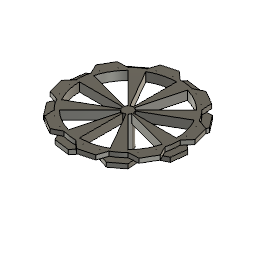
Wheel (Autodesk Fusion 360 design; units mm, degrees)
Autodesk Fusion 360 part; units mm, degrees
sketch "Sketch1" plane through (0, 0, 0) normal (0, 0, 1) x (1, 0, 0)
  circle A0 centre (0, 0) radius 35
  circle A1 centre (0, 0) radius 3.5
  line L0 (0, 0) -> (0, 35)
  line L1 (0, 0) -> (9.0587, 33.8074)
  line L2 (0, 0) -> (35, 0) construction
  line L3 (0, 35) -> (0, 40)
  line L4 (9.0587, 33.8074) -> (10.3528, 38.637)
  line L5 (10.3528, 38.637) -> (0, 40)
  line L6 (-20, 34.641) -> (-28.2843, 28.2843)
  line L7 (-24.7487, 24.7487) -> (-28.2843, 28.2843)
  line L8 (-17.5, 30.3109) -> (-20, 34.641)
  line L9 (0, 0) -> (-24.7487, 24.7487)
  line L10 (0, 0) -> (-17.5, 30.3109)
  line L11 (-38.637, 10.3528) -> (-40, 0)
  line L12 (-35, 0) -> (-40, 0)
  line L13 (-33.8074, 9.0587) -> (-38.637, 10.3528)
  line L14 (0, 0) -> (-35, 0)
  line L15 (0, 0) -> (-33.8074, 9.0587)
  line L16 (-34.641, -20) -> (-28.2843, -28.2843)
  line L17 (-24.7487, -24.7487) -> (-28.2843, -28.2843)
  line L18 (-30.3109, -17.5) -> (-34.641, -20)
  line L19 (0, 0) -> (-24.7487, -24.7487)
  line L20 (0, 0) -> (-30.3109, -17.5)
  line L21 (-10.3528, -38.637) -> (0, -40)
  line L22 (0, -35) -> (0, -40)
  line L23 (-9.0587, -33.8074) -> (-10.3528, -38.637)
  line L24 (0, 0) -> (0, -35)
  line L25 (0, 0) -> (-9.0587, -33.8074)
  line L26 (20, -34.641) -> (28.2843, -28.2843)
  line L27 (24.7487, -24.7487) -> (28.2843, -28.2843)
  line L28 (17.5, -30.3109) -> (20, -34.641)
  line L29 (0, 0) -> (24.7487, -24.7487)
  line L30 (0, 0) -> (17.5, -30.3109)
  line L31 (38.637, -10.3528) -> (40, 0)
  line L32 (35, 0) -> (40, 0)
  line L33 (33.8074, -9.0587) -> (38.637, -10.3528)
  line L34 (0, 0) -> (35, 0)
  line L35 (0, 0) -> (33.8074, -9.0587)
  line L36 (34.641, 20) -> (28.2843, 28.2843)
  line L37 (24.7487, 24.7487) -> (28.2843, 28.2843)
  line L38 (30.3109, 17.5) -> (34.641, 20)
  line L39 (0, 0) -> (24.7487, 24.7487)
  line L40 (0, 0) -> (30.3109, 17.5)
  circle A2 centre (0, 0) radius 32.5
  line L41 (38.637, -10.3528) -> (32.3341, -13.398)
  line L42 (40, 0) -> (34.7, 4.5727)
  line L43 (34.641, 20) -> (32.3375, 13.3899)
  line L44 (28.2843, 28.2843) -> (21.3032, 27.77)
  line L45 (10.3528, 38.637) -> (13.398, 32.3341)
  line L46 (0, 40) -> (-4.5727, 34.7)
  line L47 (-20, 34.641) -> (-13.3899, 32.3375)
  line L48 (-28.2843, 28.2843) -> (-27.77, 21.3032)
  line L49 (-38.637, 10.3528) -> (-32.3341, 13.398)
  line L50 (-40, 0) -> (-34.7, -4.5727)
  line L51 (-34.641, -20) -> (-32.3375, -13.3899)
  line L52 (-28.2843, -28.2843) -> (-21.3032, -27.77)
  line L53 (-10.3528, -38.637) -> (-13.398, -32.3341)
  line L54 (0, -40) -> (4.5727, -34.7)
  line L55 (20, -34.641) -> (13.3899, -32.3375)
  line L56 (28.2843, -28.2843) -> (27.77, -21.3032)
  line L57 (0, 0) -> (13.3939, -32.3358)
  line L58 (0, 0) -> (4.5684, -34.7006)
  line L59 (5.221, -39.6578) -> (15.3073, -36.9552)
  line L60 (15.3073, -36.9552) -> (17.5038, -30.3087)
  line L61 (5.221, -39.6578) -> (-0.0044, -35)
  line L62 (4.5684, -34.7006) -> (5.221, -39.6578)
  line L63 (13.3939, -32.3358) -> (15.3073, -36.9552)
  line L64 (0, 0) -> (24.7487, -24.7487)
  line L65 (0, 0) -> (17.5, -30.3109)
  line L66 (20, -34.641) -> (28.2843, -28.2843)
  line L67 (28.2843, -28.2843) -> (27.77, -21.3032)
  line L68 (20, -34.641) -> (13.3899, -32.3375)
  line L69 (17.5, -30.3109) -> (20, -34.641)
  line L70 (24.7487, -24.7487) -> (28.2843, -28.2843)
  line L71 (0, 0) -> (32.3358, -13.3939)
  line L72 (0, 0) -> (27.7674, -21.3067)
  line L73 (31.7341, -24.3505) -> (36.9552, -15.3073)
  line L74 (36.9552, -15.3073) -> (33.8085, -9.0544)
  line L75 (31.7341, -24.3505) -> (24.7456, -24.7518)
  line L76 (27.7674, -21.3067) -> (31.7341, -24.3505)
  line L77 (32.3358, -13.3939) -> (36.9552, -15.3073)
  line L78 (0, 0) -> (35, 0)
  line L79 (0, 0) -> (33.8074, -9.0587)
  line L80 (38.637, -10.3528) -> (40, 0)
  line L81 (40, 0) -> (34.7, 4.5727)
  line L82 (38.637, -10.3528) -> (32.3341, -13.398)
  line L83 (33.8074, -9.0587) -> (38.637, -10.3528)
  line L84 (35, 0) -> (40, 0)
  line L85 (0, 0) -> (32.3358, 13.3939)
  line L86 (0, 0) -> (34.7006, 4.5684)
  line L87 (39.6578, 5.221) -> (36.9552, 15.3073)
  line L88 (36.9552, 15.3073) -> (30.3087, 17.5038)
  line L89 (39.6578, 5.221) -> (35, -0.0044)
  line L90 (34.7006, 4.5684) -> (39.6578, 5.221)
  line L91 (32.3358, 13.3939) -> (36.9552, 15.3073)
  line L92 (0, 0) -> (24.7487, 24.7487)
  line L93 (0, 0) -> (30.3109, 17.5)
  line L94 (34.641, 20) -> (28.2843, 28.2843)
  line L95 (28.2843, 28.2843) -> (21.3032, 27.77)
  line L96 (34.641, 20) -> (32.3375, 13.3899)
  line L97 (30.3109, 17.5) -> (34.641, 20)
  line L98 (24.7487, 24.7487) -> (28.2843, 28.2843)
  line L99 (0, 0) -> (13.3939, 32.3358)
  line L100 (0, 0) -> (21.3067, 27.7674)
  line L101 (24.3505, 31.7341) -> (15.3073, 36.9552)
  line L102 (15.3073, 36.9552) -> (9.0544, 33.8085)
  line L103 (24.3505, 31.7341) -> (24.7518, 24.7456)
  line L104 (21.3067, 27.7674) -> (24.3505, 31.7341)
  line L105 (13.3939, 32.3358) -> (15.3073, 36.9552)
  line L106 (0, 0) -> (0, 35)
  line L107 (0, 0) -> (9.0587, 33.8074)
  line L108 (10.3528, 38.637) -> (0, 40)
  line L109 (0, 40) -> (-4.5727, 34.7)
  line L110 (10.3528, 38.637) -> (13.398, 32.3341)
  line L111 (9.0587, 33.8074) -> (10.3528, 38.637)
  line L112 (0, 35) -> (0, 40)
  line L113 (0, 0) -> (-13.3939, 32.3358)
  line L114 (0, 0) -> (-4.5684, 34.7006)
  line L115 (-5.221, 39.6578) -> (-15.3073, 36.9552)
  line L116 (-15.3073, 36.9552) -> (-17.5038, 30.3087)
  line L117 (-5.221, 39.6578) -> (0.0044, 35)
  line L118 (-4.5684, 34.7006) -> (-5.221, 39.6578)
  line L119 (-13.3939, 32.3358) -> (-15.3073, 36.9552)
  line L120 (0, 0) -> (-24.7487, 24.7487)
  line L121 (0, 0) -> (-17.5, 30.3109)
  line L122 (-20, 34.641) -> (-28.2843, 28.2843)
  line L123 (-28.2843, 28.2843) -> (-27.77, 21.3032)
  line L124 (-20, 34.641) -> (-13.3899, 32.3375)
  line L125 (-17.5, 30.3109) -> (-20, 34.641)
  line L126 (-24.7487, 24.7487) -> (-28.2843, 28.2843)
  line L127 (0, 0) -> (-32.3358, 13.3939)
  line L128 (0, 0) -> (-27.7674, 21.3067)
  line L129 (-31.7341, 24.3505) -> (-36.9552, 15.3073)
  line L130 (-36.9552, 15.3073) -> (-33.8085, 9.0544)
  line L131 (-31.7341, 24.3505) -> (-24.7456, 24.7518)
  line L132 (-27.7674, 21.3067) -> (-31.7341, 24.3505)
  line L133 (-32.3358, 13.3939) -> (-36.9552, 15.3073)
  line L134 (0, 0) -> (-35, 0)
  line L135 (0, 0) -> (-33.8074, 9.0587)
  line L136 (-38.637, 10.3528) -> (-40, 0)
  line L137 (-40, 0) -> (-34.7, -4.5727)
  line L138 (-38.637, 10.3528) -> (-32.3341, 13.398)
  line L139 (-33.8074, 9.0587) -> (-38.637, 10.3528)
  line L140 (-35, 0) -> (-40, 0)
  line L141 (0, 0) -> (-32.3358, -13.3939)
  line L142 (0, 0) -> (-34.7006, -4.5684)
  line L143 (-39.6578, -5.221) -> (-36.9552, -15.3073)
  line L144 (-36.9552, -15.3073) -> (-30.3087, -17.5038)
  line L145 (-39.6578, -5.221) -> (-35, 0.0044)
  line L146 (-34.7006, -4.5684) -> (-39.6578, -5.221)
  line L147 (-32.3358, -13.3939) -> (-36.9552, -15.3073)
  line L148 (0, 0) -> (-24.7487, -24.7487)
  line L149 (0, 0) -> (-30.3109, -17.5)
  line L150 (-34.641, -20) -> (-28.2843, -28.2843)
  line L151 (-28.2843, -28.2843) -> (-21.3032, -27.77)
  line L152 (-34.641, -20) -> (-32.3375, -13.3899)
  line L153 (-30.3109, -17.5) -> (-34.641, -20)
  line L154 (-24.7487, -24.7487) -> (-28.2843, -28.2843)
  line L155 (0, 0) -> (-13.3939, -32.3358)
  line L156 (0, 0) -> (-21.3067, -27.7674)
  line L157 (-24.3505, -31.7341) -> (-15.3073, -36.9552)
  line L158 (-15.3073, -36.9552) -> (-9.0544, -33.8085)
  line L159 (-24.3505, -31.7341) -> (-24.7518, -24.7456)
  line L160 (-21.3067, -27.7674) -> (-24.3505, -31.7341)
  line L161 (-13.3939, -32.3358) -> (-15.3073, -36.9552)
  dimension "d1" = 70
  dimension "d2" = 7
  dimension "d3" = 75
  dimension "d4" = 5
  dimension "d6" = 360
  dimension "d7" = 65
  dimension "d15" = 7
  dimension "d16" = 7
  dimension "d17" = 7
  dimension "d18" = 7
  dimension "d19" = 7
  dimension "d20" = 7
  dimension "d21" = 7
  dimension "d22" = 7
  dimension "d23" = 7
  dimension "d24" = 7
  dimension "d25" = 7
  dimension "d26" = 7
  dimension "d27" = 7
  dimension "d28" = 7
  dimension "d29" = 7
  dimension "d30" = 7
  dimension "d32" = 360
  constraint coincident A0.centre A1.centre
  constraint concentric A0 A1
  constraint coincident A0 L0.end
  constraint vertical L0
  constraint horizontal L2
  constraint parallel L0 L3
  constraint parallel L1 L4
  constraint coincident A0 L41.end
  constraint coincident A0 L42.end
  constraint coincident A0 L43.end
  constraint coincident A0 L44.end
  constraint coincident A0 L45.end
  constraint coincident A0 L46.end
  constraint coincident A0 L47.end
  constraint coincident A0 L48.end
  constraint coincident A0 L49.end
  constraint coincident A0 L50.end
  constraint coincident A0 L51.end
  constraint coincident A0 L52.end
  constraint coincident A0 L53.end
  constraint coincident A0 L54.end
  constraint coincident A0 L55.end
  constraint coincident A0 L56.end
  measures "d1" diameter of A0
  measures "d2" diameter of A1
  measures "d3" angle of L1 L2
  measures "d4" distance of L1.end L4.end
  measures "d7" diameter of A2
  measures "d15" distance of L31.start L41.end
  measures "d16" distance of L31.end L42.end
  measures "d17" distance of L36.start L43.end
  measures "d18" distance of L36.end L44.end
  measures "d19" distance of L4.end L45.end
  measures "d20" distance of L3.end L46.end
  measures "d21" distance of L6.start L47.end
  measures "d22" distance of L6.end L48.end
  measures "d23" distance of L11.start L49.end
  measures "d24" distance of L11.end L50.end
  measures "d25" distance of L16.start L51.end
  measures "d26" distance of L16.end L52.end
  measures "d27" distance of L21.start L53.end
  measures "d28" distance of L21.end L54.end
  measures "d29" distance of L26.start L55.end L0
  measures "d30" distance of L26.end L56.end
extrude "Extrude1" add sketch "Sketch1" along normal blind 5 contours A0 L34 A2 L78 L86 | A0 L32 L84 L89 | A0 L34 L35 A2 L78 L79 | A0 A2 L85 L86 | A0 L31 L32 L33 L74 L80 L83 L84 L89 | A1 L34 L35 A2 L78 L79 | A0 L33 L74 L83 | A1 L34 L78 L86 | A1 L34 L35 L78 L79 | A0 L35 A2 L71 L79 | A0 L40 A2 L85 L93 | A1 L85 L86 | A1 L35 L71 L79 | A1 L0 L106 L114 | A1 L0 L1 L106 L107 | A1 L9 L120 L128 | A1 L9 L10 L120 L121 | A1 L14 L134 L142 | A1 L14 L15 L134 L135 | A1 L19 L148 L156 | A1 L19 L20 L148 L149 | A1 L24 L58 | A1 L24 L25 | A1 L29 L64 L72 | A1 L29 L30 L64 L65 | A1 L39 L92 L100 | A1 L39 L40 L92 L93 | A1 L30 L57 L65 | A1 L57 L58 | A1 L71 L72 | A1 L40 L85 L93 | A1 L1 L99 L107 | A1 L99 L100 | A1 L10 L113 L121 | A1 L113 L114 | A1 L15 L127 L135 | A1 L127 L128 | A1 L20 L141 L149 | A1 L141 L142 | A1 L25 L155 | A1 L155 L156 | A0 A2 L71 L72 | A0 L39 L40 A2 L92 L93 | A1 L39 L40 A2 L92 L93 | A1 L0 L1 A2 L106 L107 | A1 L9 L10 A2 L120 L121 | A1 L14 L15 A2 L134 L135 | A1 L19 L20 A2 L148 L149 | A1 L24 L25 A2 | A1 L29 L30 A2 L64 L65 | A0 L29 A2 L64 L72 | A0 L38 L88 L97 | A0 L39 A2 L92 L100 | A0 L0 A2 L106 L114 | A0 L0 L1 A2 L106 L107 | A0 L1 A2 L99 L107 | A0 L9 A2 L120 L128 | A0 L9 L10 A2 L120 L121 | A0 L10 A2 L113 L121 | A0 L14 A2 L134 L142 | A0 L14 L15 A2 L134 L135 | A0 L15 A2 L127 L135 | A0 L19 A2 L148 L156 | A0 L19 L20 A2 L148 L149 | A0 L20 A2 L141 L149 | A0 L24 A2 L58 | A0 L24 L25 A2 | A0 L25 A2 L155 | A0 L29 L30 A2 L64 L65 | A0 L30 A2 L57 L65 | A0 A2 L57 L58 | A0 A2 L99 L100 | A0 A2 L113 L114 | A0 A2 L127 L128 | A0 A2 L141 L142 | A0 A2 L155 L156 | A0 L36 L37 L38 L88 L94 L97 L98 L103 | A0 L37 L98 L103 | A0 L3 L112 L117 | A0 L4 L102 L111 | A0 L7 L126 L131 | A0 L8 L116 L125 | A0 L12 L140 L145 | A0 L13 L130 L139 | A0 L17 L154 L159 | A0 L18 L144 L153 | A0 L22 L61 | A0 L23 L158 | A0 L27 L70 L75 | A0 L28 L60 L69 | A0 L3 L4 L5 L102 L108 L111 L112 L117 | A0 L6 L7 L8 L116 L122 L125 L126 L131 | A0 L11 L12 L13 L130 L136 L139 L140 L145 | A0 L16 L17 L18 L144 L150 L153 L154 L159 | A0 L21 L22 L23 L61 L158 | A0 L26 L27 L28 L60 L66 L69 L70 L75
sketch "Sketch2" plane through (0, 0, 0) normal (0, 0, -1) x (1, 0, 0)
  arc A0 (0.9059, -3.3807) -> (2.4749, -2.4749) centre (0, 0) ccw
  line L0 (2.4749, -2.4749) -> (22.981, -22.981)
  arc A1 (8.4116, -31.3926) -> (22.981, -22.981) centre (0, 0) ccw
  line L1 (8.4116, -31.3926) -> (0.9059, -3.3807)
  arc A2 (-0.9059, 3.3807) -> (-2.4749, 2.4749) centre (0, 0) ccw
  line L2 (-2.4749, 2.4749) -> (-22.981, 22.981)
  arc A3 (-8.4116, 31.3926) -> (-22.981, 22.981) centre (0, 0) ccw
  line L3 (-8.4116, 31.3926) -> (-0.9059, 3.3807)
  line L4 (3.5, 0) -> (32.5, 0)
  arc A4 (28.1458, -16.25) -> (32.5, 0) centre (0, 0) ccw
  line L5 (28.1458, -16.25) -> (3.0311, -1.75)
  arc A5 (3.0311, -1.75) -> (3.5, 0) centre (0, 0) ccw
  arc A6 (-1.75, -3.0311) -> (0, -3.5) centre (0, 0) ccw
  line L6 (0, -3.5) -> (0, -32.5)
  arc A7 (-16.25, -28.1458) -> (0, -32.5) centre (0, 0) ccw
  line L7 (-16.25, -28.1458) -> (-1.75, -3.0311)
  arc A8 (-3.0311, 1.75) -> (-3.5, 0) centre (0, 0) ccw
  line L8 (-3.5, 0) -> (-32.5, 0)
  arc A9 (-28.1458, 16.25) -> (-32.5, 0) centre (0, 0) ccw
  line L9 (-28.1458, 16.25) -> (-3.0311, 1.75)
  arc A10 (-3.3807, -0.9059) -> (-2.4749, -2.4749) centre (0, 0) ccw
  line L10 (-2.4749, -2.4749) -> (-22.981, -22.981)
  arc A11 (-31.3926, -8.4116) -> (-22.981, -22.981) centre (0, 0) ccw
  line L11 (-31.3926, -8.4116) -> (-3.3807, -0.9059)
  arc A12 (1.75, 3.0311) -> (0, 3.5) centre (0, 0) ccw
  line L12 (0, 3.5) -> (0, 32.5)
  arc A13 (16.25, 28.1458) -> (0, 32.5) centre (0, 0) ccw
  line L13 (16.25, 28.1458) -> (1.75, 3.0311)
  arc A14 (3.3807, 0.9059) -> (2.4749, 2.4749) centre (0, 0) ccw
  line L14 (2.4749, 2.4749) -> (22.981, 22.981)
  arc A15 (31.3926, 8.4116) -> (22.981, 22.981) centre (0, 0) ccw
  line L15 (31.3926, 8.4116) -> (3.3807, 0.9059)
  arc A16 (30.3109, -17.5) -> (35, 0) centre (0, 0) ccw
  line L16 (35, 0) -> (40, 0)
  line L17 (40, 0) -> (38.637, 10.3528)
  line L18 (38.637, 10.3528) -> (33.8074, 9.0587)
  arc A17 (33.8074, 9.0587) -> (24.7487, 24.7487) centre (0, 0) ccw
  line L19 (24.7487, 24.7487) -> (28.2843, 28.2843)
  line L20 (28.2843, 28.2843) -> (20, 34.641)
  line L21 (20, 34.641) -> (17.5, 30.3109)
  arc A18 (17.5, 30.3109) -> (0, 35) centre (0, 0) ccw
  line L22 (0, 35) -> (0, 40)
  line L23 (0, 40) -> (-10.3528, 38.637)
  line L24 (-10.3528, 38.637) -> (-9.0587, 33.8074)
  arc A19 (-9.0587, 33.8074) -> (-24.7487, 24.7487) centre (0, 0) ccw
  line L25 (-24.7487, 24.7487) -> (-28.2843, 28.2843)
  line L26 (-28.2843, 28.2843) -> (-34.641, 20)
  line L27 (-34.641, 20) -> (-30.3109, 17.5)
  arc A20 (-30.3109, 17.5) -> (-35, 0) centre (0, 0) ccw
  line L28 (-35, 0) -> (-40, 0)
  line L29 (-40, 0) -> (-38.637, -10.3528)
  line L30 (-38.637, -10.3528) -> (-33.8074, -9.0587)
  arc A21 (-33.8074, -9.0587) -> (-24.7487, -24.7487) centre (0, 0) ccw
  line L31 (-24.7487, -24.7487) -> (-28.2843, -28.2843)
  line L32 (-28.2843, -28.2843) -> (-20, -34.641)
  line L33 (-20, -34.641) -> (-17.5, -30.3109)
  arc A22 (-17.5, -30.3109) -> (0, -35) centre (0, 0) ccw
  line L34 (0, -35) -> (0, -40)
  line L35 (0, -40) -> (10.3528, -38.637)
  line L36 (10.3528, -38.637) -> (9.0587, -33.8074)
  arc A23 (9.0587, -33.8074) -> (24.7487, -24.7487) centre (0, 0) ccw
  line L37 (24.7487, -24.7487) -> (28.2843, -28.2843)
  line L38 (28.2843, -28.2843) -> (34.641, -20)
  line L39 (34.641, -20) -> (30.3109, -17.5)
  circle A24 centre (0, 0) radius 3.5
  circle A25 centre (0, 0) radius 2.85
  line L40 (0, 0) -> (0, 1.953)
  line L41 (0, 0) -> (0, -1.953) construction
  line L42 (0, -1.953) -> (-2.0756, -1.953)
  line L43 (0, -1.953) -> (2.0756, -1.953)
  line L44 (0, 1.953) -> (-2.0756, 1.953)
  line L45 (0, 1.953) -> (2.0756, 1.953)
  dimension "d10" = 5.7
  dimension "d11" = 1.953
  dimension "d12" = 1.953
  constraint concentric A0 A24
  constraint coincident L4.start A24
  constraint concentric A24 A25
  constraint coincident A0.centre A1.centre
  constraint vertical L40
  constraint parallel L40 L41
  constraint coincident A25 L42.end
  constraint perpendicular L41 L42
  constraint coincident A25 L43.end
  constraint perpendicular L41 L43
  constraint coincident A25 L44.end
  constraint perpendicular L40 L44
  constraint coincident A25 L45.end
  constraint perpendicular L40 L45
  measures "d10" diameter of A25
  measures "d11" distance of A0.centre L40.end
  measures "d12" distance of A0.centre L41.end
extrude "Extrude2" add sketch "Sketch2" along normal blind 15 contours A0 A2 A5 A6 A8 A10 A12 A14 A24 | A25 L44 L45 | A25 L42 L43
sketch "Sketch3" plane through (0, 0, 0) normal (0, 0, -1) x (1, 0, 0)
  arc A0 (3.5, 0) -> (3.3807, 0.9059) centre (0, 0) ccw
  line L0 (3.5, 0) -> (32.5, 0)
  arc A1 (28.1458, -16.25) -> (32.5, 0) centre (0, 0) ccw
  line L1 (28.1458, -16.25) -> (3.0311, -1.75)
  arc A2 (2.4749, -2.4749) -> (3.0311, -1.75) centre (0, 0) ccw
  line L2 (2.4749, -2.4749) -> (22.981, -22.981)
  arc A3 (8.4116, -31.3926) -> (22.981, -22.981) centre (0, 0) ccw
  line L3 (8.4116, -31.3926) -> (0.9059, -3.3807)
  arc A4 (0, -3.5) -> (0.9059, -3.3807) centre (0, 0) ccw
  line L4 (0, -3.5) -> (0, -32.5)
  arc A5 (-16.25, -28.1458) -> (0, -32.5) centre (0, 0) ccw
  line L5 (-16.25, -28.1458) -> (-1.75, -3.0311)
  arc A6 (-2.4749, -2.4749) -> (-1.75, -3.0311) centre (0, 0) ccw
  line L6 (-2.4749, -2.4749) -> (-22.981, -22.981)
  arc A7 (-31.3926, -8.4116) -> (-22.981, -22.981) centre (0, 0) ccw
  line L7 (-31.3926, -8.4116) -> (-3.3807, -0.9059)
  arc A8 (-3.5, 0) -> (-3.3807, -0.9059) centre (0, 0) ccw
  line L8 (-3.5, 0) -> (-32.5, 0)
  arc A9 (-28.1458, 16.25) -> (-32.5, 0) centre (0, 0) ccw
  line L9 (-28.1458, 16.25) -> (-3.0311, 1.75)
  arc A10 (-2.4749, 2.4749) -> (-3.0311, 1.75) centre (0, 0) ccw
  line L10 (-2.4749, 2.4749) -> (-22.981, 22.981)
  arc A11 (-8.4116, 31.3926) -> (-22.981, 22.981) centre (0, 0) ccw
  line L11 (-8.4116, 31.3926) -> (-0.9059, 3.3807)
  arc A12 (0, 3.5) -> (-0.9059, 3.3807) centre (0, 0) ccw
  line L12 (0, 3.5) -> (0, 32.5)
  arc A13 (16.25, 28.1458) -> (0, 32.5) centre (0, 0) ccw
  line L13 (16.25, 28.1458) -> (1.75, 3.0311)
  arc A14 (2.4749, 2.4749) -> (1.75, 3.0311) centre (0, 0) ccw
  line L14 (2.4749, 2.4749) -> (22.981, 22.981)
  arc A15 (31.3926, 8.4116) -> (22.981, 22.981) centre (0, 0) ccw
  line L15 (31.3926, 8.4116) -> (3.3807, 0.9059)
  arc A16 (30.3109, -17.5) -> (35, 0) centre (0, 0) ccw
  line L16 (35, 0) -> (40, 0)
  line L17 (40, 0) -> (38.637, 10.3528)
  line L18 (38.637, 10.3528) -> (33.8074, 9.0587)
  arc A17 (33.8074, 9.0587) -> (24.7487, 24.7487) centre (0, 0) ccw
  line L19 (24.7487, 24.7487) -> (28.2843, 28.2843)
  line L20 (28.2843, 28.2843) -> (20, 34.641)
  line L21 (20, 34.641) -> (17.5, 30.3109)
  arc A18 (17.5, 30.3109) -> (0, 35) centre (0, 0) ccw
  line L22 (0, 35) -> (0, 40)
  line L23 (0, 40) -> (-10.3528, 38.637)
  line L24 (-10.3528, 38.637) -> (-9.0587, 33.8074)
  arc A19 (-9.0587, 33.8074) -> (-24.7487, 24.7487) centre (0, 0) ccw
  line L25 (-24.7487, 24.7487) -> (-28.2843, 28.2843)
  line L26 (-28.2843, 28.2843) -> (-34.641, 20)
  line L27 (-34.641, 20) -> (-30.3109, 17.5)
  arc A20 (-30.3109, 17.5) -> (-35, 0) centre (0, 0) ccw
  line L28 (-35, 0) -> (-40, 0)
  line L29 (-40, 0) -> (-38.637, -10.3528)
  line L30 (-38.637, -10.3528) -> (-33.8074, -9.0587)
  arc A21 (-33.8074, -9.0587) -> (-24.7487, -24.7487) centre (0, 0) ccw
  line L31 (-24.7487, -24.7487) -> (-28.2843, -28.2843)
  line L32 (-28.2843, -28.2843) -> (-20, -34.641)
  line L33 (-20, -34.641) -> (-17.5, -30.3109)
  arc A22 (-17.5, -30.3109) -> (0, -35) centre (0, 0) ccw
  line L34 (0, -35) -> (0, -40)
  line L35 (0, -40) -> (10.3528, -38.637)
  line L36 (10.3528, -38.637) -> (9.0587, -33.8074)
  arc A23 (9.0587, -33.8074) -> (24.7487, -24.7487) centre (0, 0) ccw
  line L37 (24.7487, -24.7487) -> (28.2843, -28.2843)
  line L38 (28.2843, -28.2843) -> (34.641, -20)
  line L39 (34.641, -20) -> (30.3109, -17.5)
extrude "Extrude3" add sketch "Sketch1" along normal blind 3 contours A0 L32 L42 L81 L84 L89 L90 | L32 L42 L81 L84 L89 | A0 L33 L41 L74 L77 L82 L83 | L33 L41 L74 L82 L83 | A0 L38 L43 L88 L91 L96 L97 | L38 L43 L88 L96 L97 | A0 L27 L56 L67 L70 L75 L76 | A0 L37 L44 L95 L98 L103 L104 | A0 L3 L46 L109 L112 L117 L118 | A0 L4 L45 L102 L105 L110 L111 | A0 L7 L48 L123 L126 L131 L132 | A0 L8 L47 L116 L119 L124 L125 | A0 L12 L50 L137 L140 L145 L146 | A0 L13 L49 L130 L133 L138 L139 | A0 L17 L52 L151 L154 L159 L160 | A0 L18 L51 L144 L147 L152 L153 | A0 L22 L54 L61 L62 | A0 L23 L53 L158 L161 | A0 L28 L55 L60 L63 L68 L69 | L37 L44 L95 L98 L103 | L27 L56 L67 L70 L75 | L3 L46 L109 L112 L117 | L4 L45 L102 L110 L111 | L7 L48 L123 L126 L131 | L8 L47 L116 L124 L125 | L12 L50 L137 L140 L145 | L13 L49 L130 L138 L139 | L17 L52 L151 L154 L159 | L18 L51 L144 L152 L153 | L22 L54 L61 | L23 L53 L158 | L28 L55 L60 L68 L69
extrude "Extrude4" cut 1 faces at (13.6603, -18.0526, 5) along direction (0, 0, -1) blind 2
extrude "Extrude5" add sketch "Sketch1" along normal blind 3 from surface at 3 contours A0 L32 L42 L81 L84 L89 L90 | A0 L42 L43 L81 L87 L90 L91 L96 | A1 A2 L85 L86 | L42 L81 L89 L90 | A1 L34 L78 L86 | A1 L34 L35 L78 L79 | A1 L85 L86 | A0 L33 L41 L74 L77 L82 L83 | A1 L35 L71 L79 | A1 L0 L106 L114 | A1 L0 L1 L106 L107 | A1 L9 L120 L128 | A1 L9 L10 L120 L121 | A1 L14 L134 L142 | A1 L14 L15 L134 L135 | A1 L19 L148 L156 | A1 L19 L20 L148 L149 | A1 L24 L58 | A1 L24 L25 | A1 L29 L64 L72 | A1 L29 L30 L64 L65 | A1 L39 L92 L100 | A1 L39 L40 L92 L93 | A1 L30 L57 L65 | A1 L57 L58 | A1 L71 L72 | A1 L40 L85 L93 | A1 L1 L99 L107 | A1 L99 L100 | A1 L10 L113 L121 | A1 L113 L114 | A1 L15 L127 L135 | A1 L127 L128 | A1 L20 L141 L149 | A1 L141 L142 | A1 L25 L155 | A1 L155 L156 | A0 A2 L71 L72 | A1 A2 L71 L72 | A0 L38 L43 L88 L91 L96 L97 | L43 L88 L91 L96 | L41 L74 L77 L82 | A1 A2 L57 L58 | A1 A2 L99 L100 | A1 A2 L113 L114 | A1 A2 L127 L128 | A1 A2 L141 L142 | A1 A2 L155 L156 | A0 L41 L56 L67 L73 L76 L77 L82 | A0 A2 L57 L58 | A0 A2 L113 L114 | A0 A2 L127 L128 | A0 A2 L141 L142 | A0 A2 L155 L156 | A0 L27 L56 L67 L70 L75 L76 | A0 L37 L44 L95 L98 L103 L104 | L56 L67 L75 L76 | A0 L3 L46 L109 L112 L117 L118 | A0 L4 L45 L102 L105 L110 L111 | A0 L7 L48 L123 L126 L131 L132 | A0 L8 L47 L116 L119 L124 L125 | A0 L12 L50 L137 L140 L145 L146 | A0 L13 L49 L130 L133 L138 L139 | A0 L17 L52 L151 L154 L159 L160 | A0 L18 L51 L144 L147 L152 L153 | A0 L22 L54 L61 L62 | A0 L23 L53 L158 L161 | A0 L28 L55 L60 L63 L68 L69 | A0 L54 L55 L59 L62 L63 L68 | L55 L60 L63 L68 | L54 L61 L62 | A0 L44 L45 L95 L101 L104 L105 L110 | L45 L102 L105 L110 | L44 L95 L103 L104 | A0 L46 L47 L109 L115 L118 L119 L124 | L47 L116 L119 L124 | L46 L109 L117 L118 | A0 L48 L49 L123 L129 L132 L133 L138 | L49 L130 L133 L138 | L48 L123 L131 L132 | A0 L50 L51 L137 L143 L146 L147 L152 | L51 L144 L147 L152 | L50 L137 L145 L146 | A0 L52 L53 L151 L157 L160 L161 | L53 L158 L161 | L52 L151 L159 L160
extrude "Extrude6" add sketch "Sketch1" along normal blind 7 contours A0 A2 L85 L86 | A0 A2 L99 L100
extrude "Extrude7" cut 2 faces at (19.9656, 27.69, 7) (33.6976, 5.462, 7) along direction (0, 0, -1) blind 1
extrude "Extrude8" add sketch "Sketch1" along normal blind 3 from surface at 3 contours A0 L34 A2 L78 L86 | A0 L34 L35 A2 L78 L79 | A0 A2 L85 L86 | A0 L35 A2 L71 L79 | A0 L40 A2 L85 L93 | A0 A2 L71 L72 | A0 L39 L40 A2 L92 L93 | A0 L29 A2 L64 L72 | A0 L39 A2 L92 L100 | A0 L0 A2 L106 L114 | A0 L0 L1 A2 L106 L107 | A0 L1 A2 L99 L107 | A0 L9 A2 L120 L128 | A0 L9 L10 A2 L120 L121 | A0 L10 A2 L113 L121 | A0 L14 A2 L134 L142 | A0 L14 L15 A2 L134 L135 | A0 L15 A2 L127 L135 | A0 L19 A2 L148 L156 | A0 L19 L20 A2 L148 L149 | A0 L20 A2 L141 L149 | A0 L24 A2 L58 | A0 L24 L25 A2 | A0 L25 A2 L155 | A0 L29 L30 A2 L64 L65 | A0 L30 A2 L57 L65 | A0 A2 L57 L58 | A0 A2 L99 L100 | A0 A2 L113 L114 | A0 A2 L127 L128 | A0 A2 L141 L142 | A0 A2 L155 L156
extrude "Extrude9" add 8 faces at (22.2819, -4.8877, 3) (16.8529, 15.3738, 3) (15.4488, -16.7841, 3) (-4.8877, -22.2819, 3) (-18.0667, -13.9272, 3) (-22.7921, 0.9442, 3) (-13.9272, 18.0667, 3) (2.9271, 22.6231, 3) along direction (0, 0, 1) blind 3
extrude "Extrude10" cut 8 faces at (-22.4562, -4.0113, 3) (-9.6867, -20.6528, 3) (4.0113, -22.4562, 3) (19.73, -11.4499, 3) (22.0211, 5.9532, 3) (11.4499, 19.73, 3) (-4.0113, 22.4562, 3) (-20.6528, 9.6867, 3) along direction (0, 0, 1) blind 3
equation "d49 = 0 mm - 3 mm"
